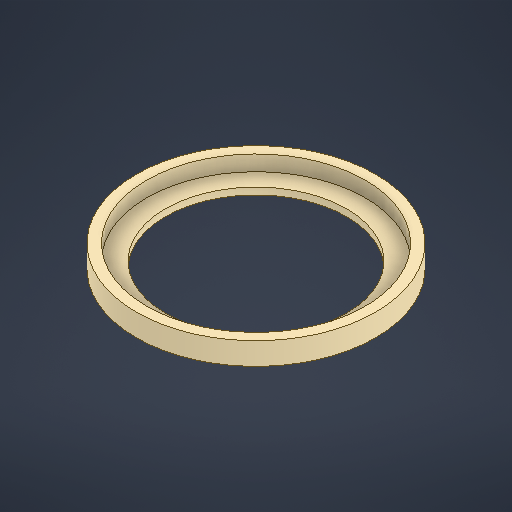
# Autodesk Inventor part: GFK_Unterlegring
Saved by Autodesk Inventor 2027 (Build 310192060, 192F)
## iProperties
Created: 2026-07-31
Part Number: GFK_Unterlegring
Material: Default New Material
Document SubType Name: Modeling
Designer: kw
Density: 1 g/cm^3
Appearance: Generic
Author: kw
Autodesk Inventor part; units mm, degrees
ref_plane "YZ Plane" through (0, 0, 0) normal (1, 0, 0) x (0, 1, 0)
ref_plane "XZ Plane" through (0, 0, 0) normal (0, 1, 0) x (-1, 0, 0)
ref_plane "XY Plane" through (0, 0, 0) normal (0, 0, 1) x (1, 0, 0)
sketch "Sketch1" plane through (0, 0, 0) normal (0, 1, 0) x (-1, 0, 0)
  circle A0 centre (0, 0) radius 32
  circle A1 centre (0, 0) radius 41.5
  circle A2 centre (0, 0) radius 35
  circle A3 centre (0, 0) radius 26.5
  dimension "d0" = 64
  dimension "d1" = 83
  dimension "d2" = 3
  dimension "d5" = 53
  constraints: 4 centre point, 3 coincident
  measures "d0" diameter of A0
  measures "d1" diameter of A1
  measures "d2" radial gap between concentric circles of A0 A2
  measures "d5" diameter of A3
extrude "Extrusion1" add sketch "Sketch1" along normal blind 2 contours A0
extrude "Extrusion2" add sketch "Sketch1" along normal blind 6.5 contours A2
body "Solid1"
